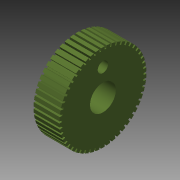
# Autodesk Inventor part: driverwheel
Saved by Autodesk Inventor 2015 (Build 190159000, 159)
## iProperties
Created: 2020-01-20
Part Number: driverwheel
Material: Aluminum 6061-AHC
Document SubType Name: Modeling
Designer: hp
Density: 2.7 g/cm^3
Appearance: Aluminum - Dark
Author: hp
Autodesk Inventor part; units mm, degrees
ref_plane "YZ Plane" through (0, 0, 0) normal (1, 0, 0) x (0, 1, 0)
ref_plane "XZ Plane" through (0, 0, 0) normal (0, 1, 0) x (-1, 0, 0)
ref_plane "XY Plane" through (0, 0, 0) normal (0, 0, 1) x (1, 0, 0)
sketch "Sketch1" plane through (0, 0, 0) normal (1, 0, 0) x (0, 1, 0)
  circle A0 centre (0, 0) radius 199.9996
  circle A1 centre (0, 0) radius 63.5
  line L0 (213.1358, 8.3999) -> (194.8022, 8.3999)
  line L1 (194.8022, 8.3999) -> (194.8022, -8.9864)
  line L2 (194.8022, -8.9864) -> (213.1358, -8.9864)
  line L3 (213.1358, -8.9864) -> (213.1358, 8.3999)
  line L4 (212.508, -18.3793) -> (194.3189, -16.0815)
  line L5 (194.3189, -16.0815) -> (192.1398, -33.3307)
  line L6 (192.1398, -33.3307) -> (210.3289, -35.6285)
  line L7 (210.3289, -35.6285) -> (212.508, -18.3793)
  line L8 (208.5287, -44.8687) -> (190.7711, -40.3093)
  line L9 (190.7711, -40.3093) -> (186.4473, -57.1494)
  line L10 (186.4473, -57.1494) -> (204.2049, -61.7088)
  line L11 (204.2049, -61.7088) -> (208.5287, -44.8687)
  line L12 (201.2609, -70.6505) -> (184.2147, -63.9014)
  line L13 (184.2147, -63.9014) -> (177.8144, -80.0668)
  line L14 (177.8144, -80.0668) -> (194.8606, -86.8159)
  line L15 (194.8606, -86.8159) -> (201.2609, -70.6505)
  line L16 (190.819, -95.3181) -> (174.7531, -86.4858)
  line L17 (174.7531, -86.4858) -> (166.3772, -101.7215)
  line L18 (166.3772, -101.7215) -> (182.4431, -110.5538)
  line L19 (182.4431, -110.5538) -> (190.819, -95.3181)
  line L20 (177.3678, -118.4824) -> (162.5356, -107.7062)
  line L21 (162.5356, -107.7062) -> (152.3162, -121.772)
  line L22 (152.3162, -121.772) -> (167.1484, -132.5482)
  line L23 (167.1484, -132.5482) -> (177.3678, -118.4824)
  line L24 (161.1194, -139.7782) -> (147.7548, -127.228)
  line L25 (147.7548, -127.228) -> (135.8531, -139.9021)
  line L26 (135.8531, -139.9021) -> (149.2177, -152.4523)
  line L27 (149.2177, -152.4523) -> (161.1194, -139.7782)
  line L28 (142.3301, -158.8697) -> (130.6438, -144.7434)
  line L29 (130.6438, -144.7434) -> (117.2475, -155.8258)
  line L30 (117.2475, -155.8258) -> (128.9338, -169.9521)
  line L31 (128.9338, -169.9521) -> (142.3301, -158.8697)
  line L32 (121.2961, -175.4556) -> (111.4725, -159.976)
  line L33 (111.4725, -159.976) -> (96.7928, -169.2921)
  line L34 (96.7928, -169.2921) -> (106.6164, -184.7717)
  line L35 (106.6164, -184.7717) -> (121.2961, -175.4556)
  line L36 (98.3493, -189.2745) -> (90.5432, -172.6858)
  line L37 (90.5432, -172.6858) -> (74.8116, -180.0885)
  line L38 (74.8116, -180.0885) -> (82.6177, -196.6773)
  line L39 (82.6177, -196.6773) -> (98.3493, -189.2745)
  line L40 (73.8514, -200.1085) -> (68.186, -182.6722)
  line L41 (68.186, -182.6722) -> (51.6506, -188.0448)
  line L42 (51.6506, -188.0448) -> (57.316, -205.4811)
  line L43 (57.316, -205.4811) -> (73.8514, -200.1085)
  line L44 (48.1888, -207.7866) -> (44.7534, -189.7777)
  line L45 (44.7534, -189.7777) -> (27.6751, -193.0356)
  line L46 (27.6751, -193.0356) -> (31.1105, -211.0445)
  line L47 (31.1105, -211.0445) -> (48.1888, -207.7866)
  line L48 (21.7662, -212.1878) -> (20.615, -193.8903)
  line L49 (20.615, -193.8903) -> (3.2631, -194.982)
  line L50 (3.2631, -194.982) -> (4.4143, -213.2795)
  line L51 (4.4143, -213.2795) -> (21.7662, -212.1878)
  line L52 (-4.9996, -213.2427) -> (-3.8484, -194.9452)
  line L53 (-3.8484, -194.9452) -> (-21.2004, -193.8535)
  line L54 (-21.2004, -193.8535) -> (-22.3516, -212.151)
  line L55 (-22.3516, -212.151) -> (-4.9996, -213.2427)
  line L56 (-31.6866, -210.9346) -> (-28.2512, -192.9257)
  line L57 (-28.2512, -192.9257) -> (-45.3295, -189.6678)
  line L58 (-45.3295, -189.6678) -> (-48.7649, -207.6767)
  line L59 (-48.7649, -207.6767) -> (-31.6866, -210.9346)
  line L60 (-57.8738, -205.2999) -> (-52.2084, -187.8636)
  line L61 (-52.2084, -187.8636) -> (-68.7437, -182.4909)
  line L62 (-68.7437, -182.4909) -> (-74.4091, -199.9273)
  line L63 (-74.4091, -199.9273) -> (-57.8738, -205.2999)
  line L64 (-83.1484, -196.4275) -> (-75.3423, -179.8388)
  line L65 (-75.3423, -179.8388) -> (-91.0739, -172.4361)
  line L66 (-91.0739, -172.4361) -> (-98.8799, -189.0248)
  line L67 (-98.8799, -189.0248) -> (-83.1484, -196.4275)
  line L68 (-107.1116, -184.4574) -> (-97.288, -168.9778)
  line L69 (-97.288, -168.9778) -> (-111.9677, -159.6618)
  line L70 (-111.9677, -159.6618) -> (-121.7913, -175.1414)
  line L71 (-121.7913, -175.1414) -> (-107.1116, -184.4574)
  line L72 (-129.3857, -169.5783) -> (-117.6994, -155.4519)
  line L73 (-117.6994, -155.4519) -> (-131.0957, -144.3695)
  line L74 (-131.0957, -144.3695) -> (-142.782, -158.4958)
  line L75 (-142.782, -158.4958) -> (-129.3857, -169.5783)
  line L76 (-149.6192, -152.0248) -> (-136.2546, -139.4745)
  line L77 (-136.2546, -139.4745) -> (-148.1563, -126.8005)
  line L78 (-148.1563, -126.8005) -> (-161.5209, -139.3507)
  line L79 (-161.5209, -139.3507) -> (-149.6192, -152.0248)
  line L80 (-167.4932, -132.0737) -> (-152.6609, -121.2975)
  line L81 (-152.6609, -121.2975) -> (-162.8803, -107.2317)
  line L82 (-162.8803, -107.2317) -> (-177.7126, -118.008)
  line L83 (-177.7126, -118.008) -> (-167.4932, -132.0737)
  line L84 (-182.7257, -110.0398) -> (-166.6598, -101.2075)
  line L85 (-166.6598, -101.2075) -> (-175.0357, -85.9718)
  line L86 (-175.0357, -85.9718) -> (-191.1016, -94.8041)
  line L87 (-191.1016, -94.8041) -> (-182.7257, -110.0398)
  line L88 (-195.0765, -86.2705) -> (-178.0303, -79.5215)
  line L89 (-178.0303, -79.5215) -> (-184.4306, -63.3561)
  line L90 (-184.4306, -63.3561) -> (-201.4768, -70.1052)
  line L91 (-201.4768, -70.1052) -> (-195.0765, -86.2705)
  line L92 (-204.3508, -61.1407) -> (-186.5931, -56.5813)
  line L93 (-186.5931, -56.5813) -> (-190.9169, -39.7413)
  line L94 (-190.9169, -39.7413) -> (-208.6746, -44.3007)
  line L95 (-208.6746, -44.3007) -> (-204.3508, -61.1407)
  line L96 (-210.4024, -35.0467) -> (-192.2133, -32.7488)
  line L97 (-192.2133, -32.7488) -> (-194.3924, -15.4997)
  line L98 (-194.3924, -15.4997) -> (-212.5815, -17.7975)
  line L99 (-212.5815, -17.7975) -> (-210.4024, -35.0467)
  line L100 (-213.1358, -8.3999) -> (-194.8022, -8.3999)
  line L101 (-194.8022, -8.3999) -> (-194.8022, 8.9864)
  line L102 (-194.8022, 8.9864) -> (-213.1358, 8.9864)
  line L103 (-213.1358, 8.9864) -> (-213.1358, -8.3999)
  line L104 (-212.508, 18.3793) -> (-194.3189, 16.0815)
  line L105 (-194.3189, 16.0815) -> (-192.1398, 33.3307)
  line L106 (-192.1398, 33.3307) -> (-210.3289, 35.6285)
  line L107 (-210.3289, 35.6285) -> (-212.508, 18.3793)
  line L108 (-208.5287, 44.8687) -> (-190.7711, 40.3093)
  line L109 (-190.7711, 40.3093) -> (-186.4473, 57.1494)
  line L110 (-186.4473, 57.1494) -> (-204.2049, 61.7088)
  line L111 (-204.2049, 61.7088) -> (-208.5287, 44.8687)
  line L112 (-201.2609, 70.6505) -> (-184.2147, 63.9014)
  line L113 (-184.2147, 63.9014) -> (-177.8144, 80.0668)
  line L114 (-177.8144, 80.0668) -> (-194.8606, 86.8159)
  line L115 (-194.8606, 86.8159) -> (-201.2609, 70.6505)
  line L116 (-190.819, 95.3181) -> (-174.7531, 86.4858)
  line L117 (-174.7531, 86.4858) -> (-166.3772, 101.7215)
  line L118 (-166.3772, 101.7215) -> (-182.4431, 110.5538)
  line L119 (-182.4431, 110.5538) -> (-190.819, 95.3181)
  line L120 (-177.3678, 118.4824) -> (-162.5356, 107.7062)
  line L121 (-162.5356, 107.7062) -> (-152.3162, 121.772)
  line L122 (-152.3162, 121.772) -> (-167.1484, 132.5482)
  line L123 (-167.1484, 132.5482) -> (-177.3678, 118.4824)
  line L124 (-161.1194, 139.7782) -> (-147.7548, 127.228)
  line L125 (-147.7548, 127.228) -> (-135.8531, 139.9021)
  line L126 (-135.8531, 139.9021) -> (-149.2177, 152.4523)
  line L127 (-149.2177, 152.4523) -> (-161.1194, 139.7782)
  line L128 (-142.3301, 158.8697) -> (-130.6438, 144.7434)
  line L129 (-130.6438, 144.7434) -> (-117.2475, 155.8258)
  line L130 (-117.2475, 155.8258) -> (-128.9338, 169.9521)
  line L131 (-128.9338, 169.9521) -> (-142.3301, 158.8697)
  line L132 (-121.2961, 175.4556) -> (-111.4725, 159.976)
  line L133 (-111.4725, 159.976) -> (-96.7928, 169.2921)
  line L134 (-96.7928, 169.2921) -> (-106.6164, 184.7717)
  line L135 (-106.6164, 184.7717) -> (-121.2961, 175.4556)
  line L136 (-98.3493, 189.2745) -> (-90.5432, 172.6858)
  line L137 (-90.5432, 172.6858) -> (-74.8116, 180.0885)
  line L138 (-74.8116, 180.0885) -> (-82.6177, 196.6773)
  line L139 (-82.6177, 196.6773) -> (-98.3493, 189.2745)
  line L140 (-73.8514, 200.1085) -> (-68.186, 182.6722)
  line L141 (-68.186, 182.6722) -> (-51.6506, 188.0448)
  line L142 (-51.6506, 188.0448) -> (-57.316, 205.4811)
  line L143 (-57.316, 205.4811) -> (-73.8514, 200.1085)
  line L144 (-48.1888, 207.7866) -> (-44.7534, 189.7777)
  line L145 (-44.7534, 189.7777) -> (-27.6751, 193.0356)
  line L146 (-27.6751, 193.0356) -> (-31.1105, 211.0445)
  line L147 (-31.1105, 211.0445) -> (-48.1888, 207.7866)
  line L148 (-21.7662, 212.1878) -> (-20.615, 193.8903)
  line L149 (-20.615, 193.8903) -> (-3.2631, 194.982)
  line L150 (-3.2631, 194.982) -> (-4.4143, 213.2795)
  line L151 (-4.4143, 213.2795) -> (-21.7662, 212.1878)
  line L152 (4.9996, 213.2427) -> (3.8484, 194.9452)
  line L153 (3.8484, 194.9452) -> (21.2004, 193.8535)
  line L154 (21.2004, 193.8535) -> (22.3516, 212.151)
  line L155 (22.3516, 212.151) -> (4.9996, 213.2427)
  line L156 (31.6866, 210.9346) -> (28.2512, 192.9257)
  line L157 (28.2512, 192.9257) -> (45.3295, 189.6678)
  line L158 (45.3295, 189.6678) -> (48.7649, 207.6767)
  line L159 (48.7649, 207.6767) -> (31.6866, 210.9346)
  line L160 (57.8738, 205.2999) -> (52.2084, 187.8636)
  line L161 (52.2084, 187.8636) -> (68.7437, 182.4909)
  line L162 (68.7437, 182.4909) -> (74.4091, 199.9273)
  line L163 (74.4091, 199.9273) -> (57.8738, 205.2999)
  line L164 (83.1484, 196.4275) -> (75.3423, 179.8388)
  line L165 (75.3423, 179.8388) -> (91.0739, 172.4361)
  line L166 (91.0739, 172.4361) -> (98.8799, 189.0248)
  line L167 (98.8799, 189.0248) -> (83.1484, 196.4275)
  line L168 (107.1116, 184.4574) -> (97.288, 168.9778)
  line L169 (97.288, 168.9778) -> (111.9677, 159.6618)
  line L170 (111.9677, 159.6618) -> (121.7913, 175.1414)
  line L171 (121.7913, 175.1414) -> (107.1116, 184.4574)
  line L172 (129.3857, 169.5783) -> (117.6994, 155.4519)
  line L173 (117.6994, 155.4519) -> (131.0957, 144.3695)
  line L174 (131.0957, 144.3695) -> (142.782, 158.4958)
  line L175 (142.782, 158.4958) -> (129.3857, 169.5783)
  line L176 (149.6192, 152.0248) -> (136.2546, 139.4745)
  line L177 (136.2546, 139.4745) -> (148.1563, 126.8005)
  line L178 (148.1563, 126.8005) -> (161.5209, 139.3507)
  line L179 (161.5209, 139.3507) -> (149.6192, 152.0248)
  line L180 (167.4932, 132.0737) -> (152.6609, 121.2975)
  line L181 (152.6609, 121.2975) -> (162.8803, 107.2317)
  line L182 (162.8803, 107.2317) -> (177.7126, 118.008)
  line L183 (177.7126, 118.008) -> (167.4932, 132.0737)
  line L184 (182.7257, 110.0398) -> (166.6598, 101.2075)
  line L185 (166.6598, 101.2075) -> (175.0357, 85.9718)
  line L186 (175.0357, 85.9718) -> (191.1016, 94.8041)
  line L187 (191.1016, 94.8041) -> (182.7257, 110.0398)
  line L188 (195.0765, 86.2705) -> (178.0303, 79.5215)
  line L189 (178.0303, 79.5215) -> (184.4306, 63.3561)
  line L190 (184.4306, 63.3561) -> (201.4768, 70.1052)
  line L191 (201.4768, 70.1052) -> (195.0765, 86.2705)
  line L192 (204.3508, 61.1407) -> (186.5931, 56.5813)
  line L193 (186.5931, 56.5813) -> (190.9169, 39.7413)
  line L194 (190.9169, 39.7413) -> (208.6746, 44.3007)
  line L195 (208.6746, 44.3007) -> (204.3508, 61.1407)
  line L196 (210.4024, 35.0467) -> (192.2133, 32.7488)
  line L197 (192.2133, 32.7488) -> (194.3924, 15.4997)
  line L198 (194.3924, 15.4997) -> (212.5815, 17.7975)
  line L199 (212.5815, 17.7975) -> (210.4024, 35.0467)
  dimension "d0" = 399.9992
  dimension "d1" = 127
  dimension "d4" = 360
  constraints: 400 end point, 53 coincident, 2 centre point, 2 parallel, 1 horizontal, 1 perpendicular, 498 other
  measures "d0" diameter of A0
  measures "d1" diameter of A1
extrude "Extrusion1" add sketch "Sketch1" along normal blind 127
sketch "Sketch2" plane through (127, 0, 0) normal (1, 0, 0) x (0, 0, -1)
  circle A0 centre (0, 129.2465) radius 25.4
  point P0 (0, 0)
  dimension "d8" = 50.8
  constraints: 1 centre point
  measures "d8" diameter of A0
extrude "Extrusion2" cut sketch "Sketch2" against normal blind 254
body "Solid1"
